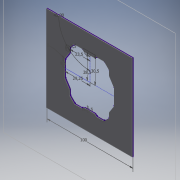
# Autodesk Inventor part: tarot_PCB_center
Saved by Autodesk Inventor 2017 (Build 210142000, 142)
## iProperties
Created: 2016-07-15
Part Number: tarot_PCB_center
Material: Generic
Document SubType Name: Modeling
Designer: Mert
Density: 1 g/cm^3
Appearance: Default
offset: 0,500 mm
PCB_thickness: 1,600 mm
Author: Mert
Autodesk Inventor part; units mm, degrees
ref_plane "YZ Plane" through (0, 0, 0) normal (1, 0, 0) x (0, 1, 0)
ref_plane "XZ Plane" through (0, 0, 0) normal (0, 1, 0) x (-1, 0, 0)
ref_plane "XY Plane" through (0, 0, 0) normal (0, 0, 1) x (1, 0, 0)
sketch "Sketch1" plane through (0, 0, 0) normal (0, 1, 0) x (-1, 0, 0)
  line L0 (0, 0) -> (0, 28.5) construction
  line L1 (0, 28.5) -> (5.5858, 28.5) construction
  line L2 (6.2929, 28.7929) -> (7.7071, 30.2071) construction
  line L3 (8.4142, 30.5) -> (17.0754, 30.5) construction
  line L4 (17.7825, 30.2071) -> (23.2071, 24.7825) construction
  line L5 (23.5, 24.0754) -> (23.5, 18.7821) construction
  line L6 (23.6576, 18.2432) -> (29.0924, 9.7464) construction
  line L7 (29.25, 9.2075) -> (29.25, 0) construction
  line L8 (29.25, 0) -> (0, 0) construction
  arc A0 (29.25, 9.2075) -> (29.0924, 9.7464) centre (28.25, 9.2075) ccw construction
  arc A1 (23.5, 18.7821) -> (23.6576, 18.2432) centre (24.5, 18.7821) ccw construction
  arc A2 (23.5, 24.0754) -> (23.2071, 24.7825) centre (22.5, 24.0754) ccw construction
  arc A3 (17.7825, 30.2071) -> (17.0754, 30.5) centre (17.0754, 29.5) ccw construction
  arc A4 (8.4142, 30.5) -> (7.7071, 30.2071) centre (8.4142, 29.5) ccw construction
  arc A5 (5.5858, 28.5) -> (6.2929, 28.7929) centre (5.5858, 29.5) ccw construction
  line L9 (0, 28.5) -> (-5.5858, 28.5) construction
  line L10 (-6.2929, 28.7929) -> (-7.7071, 30.2071) construction
  line L11 (-8.4142, 30.5) -> (-17.0754, 30.5) construction
  line L12 (-17.7825, 30.2071) -> (-23.2071, 24.7825) construction
  line L13 (-23.5, 24.0754) -> (-23.5, 18.7821) construction
  line L14 (-23.6576, 18.2432) -> (-29.0924, 9.7464) construction
  line L15 (-29.25, 9.2075) -> (-29.25, 0) construction
  arc A6 (-29.0924, 9.7464) -> (-29.25, 9.2075) centre (-28.25, 9.2075) ccw construction
  arc A7 (-23.6576, 18.2432) -> (-23.5, 18.7821) centre (-24.5, 18.7821) ccw construction
  arc A8 (-23.2071, 24.7825) -> (-23.5, 24.0754) centre (-22.5, 24.0754) ccw construction
  arc A9 (-17.0754, 30.5) -> (-17.7825, 30.2071) centre (-17.0754, 29.5) ccw construction
  arc A10 (-7.7071, 30.2071) -> (-8.4142, 30.5) centre (-8.4142, 29.5) ccw construction
  arc A11 (-6.2929, 28.7929) -> (-5.5858, 28.5) centre (-5.5858, 29.5) ccw construction
  line L16 (0, -28.5) -> (5.5858, -28.5) construction
  line L17 (6.2929, -28.7929) -> (7.7071, -30.2071) construction
  line L18 (8.4142, -30.5) -> (17.0754, -30.5) construction
  line L19 (17.7825, -30.2071) -> (23.2071, -24.7825) construction
  line L20 (23.5, -24.0754) -> (23.5, -18.7821) construction
  line L21 (23.6576, -18.2432) -> (29.0924, -9.7464) construction
  line L22 (29.25, -9.2075) -> (29.25, 0) construction
  arc A12 (29.0924, -9.7464) -> (29.25, -9.2075) centre (28.25, -9.2075) ccw construction
  arc A13 (23.6576, -18.2432) -> (23.5, -18.7821) centre (24.5, -18.7821) ccw construction
  arc A14 (23.2071, -24.7825) -> (23.5, -24.0754) centre (22.5, -24.0754) ccw construction
  arc A15 (17.0754, -30.5) -> (17.7825, -30.2071) centre (17.0754, -29.5) ccw construction
  arc A16 (7.7071, -30.2071) -> (8.4142, -30.5) centre (8.4142, -29.5) ccw construction
  arc A17 (6.2929, -28.7929) -> (5.5858, -28.5) centre (5.5858, -29.5) ccw construction
  arc A18 (-23.5, -18.7821) -> (-23.6576, -18.2432) centre (-24.5, -18.7821) ccw construction
  line L23 (-23.6576, -18.2432) -> (-29.0924, -9.7464) construction
  arc A19 (-29.25, -9.2075) -> (-29.0924, -9.7464) centre (-28.25, -9.2075) ccw construction
  line L24 (-29.25, -9.2075) -> (-29.25, 0) construction
  line L25 (0, -28.5) -> (-5.5858, -28.5) construction
  line L26 (-6.2929, -28.7929) -> (-7.7071, -30.2071) construction
  line L27 (-8.4142, -30.5) -> (-17.0754, -30.5) construction
  line L28 (-23.5, -24.0754) -> (-23.5, -18.7821) construction
  arc A20 (-23.5, -24.0754) -> (-23.2071, -24.7825) centre (-22.5, -24.0754) ccw construction
  line L29 (-17.7825, -30.2071) -> (-23.2071, -24.7825) construction
  arc A21 (-17.7825, -30.2071) -> (-17.0754, -30.5) centre (-17.0754, -29.5) ccw construction
  arc A22 (-5.5858, -28.5) -> (-6.2929, -28.7929) centre (-5.5858, -29.5) ccw construction
  arc A23 (-8.4142, -30.5) -> (-7.7071, -30.2071) centre (-8.4142, -29.5) ccw construction
  line L30 (5.5858, -28) -> (0, -28)
  line L31 (0, -28) -> (-5.5858, -28)
  arc A24 (-5.5858, -28) -> (-6.6464, -28.4393) centre (-5.5858, -29.5) ccw
  line L32 (-6.6464, -28.4393) -> (-8.2071, -30)
  line L33 (-8.2071, -30) -> (-17.2825, -30)
  line L34 (-17.2825, -30) -> (-23, -24.2825)
  line L35 (-23, -24.2825) -> (-23, -18.7821)
  arc A25 (-23, -18.7821) -> (-23.2364, -17.9738) centre (-24.5, -18.7821) ccw
  line L36 (-23.2364, -17.9738) -> (-28.75, -9.3538)
  line L37 (-28.75, -9.3538) -> (-28.75, 0)
  line L38 (-28.75, 0) -> (-28.75, 9.3538)
  line L39 (-28.75, 9.3538) -> (-23.2364, 17.9738)
  arc A26 (-23.2364, 17.9738) -> (-23, 18.7821) centre (-24.5, 18.7821) ccw
  line L40 (-23, 18.7821) -> (-23, 24.2825)
  line L41 (-23, 24.2825) -> (-17.2825, 30)
  line L42 (-17.2825, 30) -> (-8.2071, 30)
  line L43 (-8.2071, 30) -> (-6.6464, 28.4393)
  arc A27 (-6.6464, 28.4393) -> (-5.5858, 28) centre (-5.5858, 29.5) ccw
  line L44 (-5.5858, 28) -> (0, 28)
  line L45 (0, 28) -> (5.5858, 28)
  arc A28 (5.5858, 28) -> (6.6464, 28.4393) centre (5.5858, 29.5) ccw
  line L46 (6.6464, 28.4393) -> (8.2071, 30)
  line L47 (8.2071, 30) -> (17.2825, 30)
  line L48 (17.2825, 30) -> (23, 24.2825)
  line L49 (23, 24.2825) -> (23, 18.7821)
  arc A29 (23, 18.7821) -> (23.2364, 17.9738) centre (24.5, 18.7821) ccw
  line L50 (23.2364, 17.9738) -> (28.75, 9.3538)
  line L51 (28.75, 9.3538) -> (28.75, 0)
  line L52 (28.75, 0) -> (28.75, -9.3538)
  line L53 (28.75, -9.3538) -> (23.2364, -17.9738)
  arc A30 (23.2364, -17.9738) -> (23, -18.7821) centre (24.5, -18.7821) ccw
  line L54 (23, -18.7821) -> (23, -24.2825)
  line L55 (23, -24.2825) -> (17.2825, -30)
  line L56 (17.2825, -30) -> (8.2071, -30)
  line L57 (8.2071, -30) -> (6.6464, -28.4393)
  arc A31 (6.6464, -28.4393) -> (5.5858, -28) centre (5.5858, -29.5) ccw
  line L58 (-50, 50) -> (50, 50)
  line L59 (50, 50) -> (50, -50)
  line L60 (50, -50) -> (-50, -50)
  line L61 (-50, -50) -> (-50, 50)
  line L62 (50, 0) -> (-50, 0) construction
  point P0 (6, 28.5)
  point P1 (17.4896, 30.5)
  point P2 (23.5, 24.4896)
  point P3 (23.5, 18.4896)
  point P4 (29.25, 9.5)
  point P5 (-6, 28.5)
  point P6 (-17.4896, 30.5)
  point P7 (-23.5, 24.4896)
  point P8 (-23.5, 18.4896)
  point P9 (-29.25, 9.5)
  point P10 (6, -28.5)
  point P11 (17.4896, -30.5)
  point P12 (23.5, -24.4896)
  point P13 (23.5, -18.4896)
  point P14 (29.25, -9.5)
  point P15 (-23.5, -18.4896)
  point P16 (-29.25, -9.5)
  point P17 (-6, -28.5)
  point P18 (-17.4896, -30.5)
  point P19 (-23.5, -24.4896)
  dimension "d0" = 45
  dimension "d1" = 6
  dimension "d2" = 30.5
  dimension "d3" = 28.5
  dimension "d4" = 29.25
  dimension "d5" = 6
  dimension "d6" = 9.5
  dimension "d7" = 23.5
  dimension "d8" = 8.5
  dimension "d9" = 1
  dimension "d10" = 0.5
  dimension "d11" = 100
  constraints: 126 end point, 71 symmetric about line, 64 point on circle, 40 point on line, 32 centre point, 12 tangent, 6 parallel, 6 perpendicular, 5 equal radius, 3 midpoint, 1 horizontal, 1 vertical, 53 other
  measures "d0" angle of L0 L4
  measures "d1" distance of L0.end point (6, 28.5)
  measures "d2" distance between parallel lines of L8 L3
  measures "d3" distance between parallel lines of L8 L1
  measures "d4" distance between parallel lines of L0 L7
  measures "d5" distance of point (23.5, 24.49) point (23.5, 18.49)
  measures "d6" distance of point (29.25, 9.5) L7.end
  measures "d7" distance between parallel lines of L5 L0
  measures "d8" distance of point (17.49, 30.5) point (23.5, 24.49)
  measures "d9" radius of A0
  measures "d10" distance between parallel lines of L16 L30
  measures "d11" distance of L59.end L60.end
extrude "Extrusion1" add sketch "Sketch1" along normal mid plane 1.6
equation "\"d10\" = offset"
equation "\"offset\" = 0.5"
body "Solid1"
